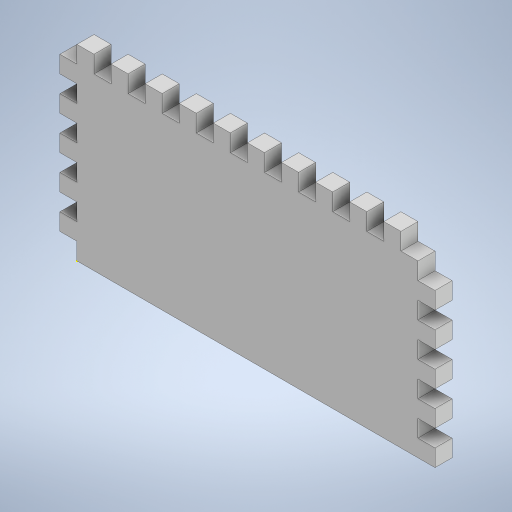
# Autodesk Inventor part: frontbackside
Saved by Autodesk Inventor 2024 (Build 280153000, 153)
## iProperties
Created: 2024-04-15
Part Number: frontbackside
Material: Generic
Document SubType Name: Modeling
Designer: srika
Density: 1 g/cm^3
Appearance: Default
Author: srika
Autodesk Inventor part; units mm, degrees
ref_plane "YZ Plane" through (0, 0, 0) normal (1, 0, 0) x (0, 1, 0)
ref_plane "XZ Plane" through (0, 0, 0) normal (0, 1, 0) x (-1, 0, 0)
ref_plane "XY Plane" through (0, 0, 0) normal (0, 0, 1) x (1, 0, 0)
sketch "Sketch1" plane through (0, 0, 0) normal (0, 0, 1) x (1, 0, 0)
  point P0 (0, 0)
sketch "Sketch2" plane through (0, 0, 0) normal (0, 0, 1) x (1, 0, 0)
  line L0 (0, 0) -> (5, 0)
  line L1 (5, 0) -> (5, 5)
  line L2 (5, 5) -> (0, 5)
  line L3 (0, 5) -> (0, 0)
  line L4 (5, 5) -> (105, 5)
  line L5 (105, 5) -> (105, 55)
  line L6 (105, 55) -> (5, 55)
  line L7 (5, 55) -> (5, 5)
  line L8 (105, 55) -> (110, 55)
  line L9 (110, 55) -> (110, 60)
  line L10 (110, 60) -> (105, 60)
  line L11 (105, 60) -> (105, 55)
  line L12 (100, 60) -> (95, 60)
  line L13 (100, 55) -> (100, 60)
  line L14 (95, 60) -> (95, 55)
  line L15 (90, 60) -> (85, 60)
  line L16 (90, 55) -> (90, 60)
  line L17 (85, 60) -> (85, 55)
  line L18 (80, 60) -> (75, 60)
  line L19 (80, 55) -> (80, 60)
  line L20 (75, 60) -> (75, 55)
  line L21 (70, 60) -> (65, 60)
  line L22 (70, 55) -> (70, 60)
  line L23 (65, 60) -> (65, 55)
  line L24 (60, 60) -> (55, 60)
  line L25 (60, 55) -> (60, 60)
  line L26 (55, 60) -> (55, 55)
  line L27 (50, 60) -> (45, 60)
  line L28 (50, 55) -> (50, 60)
  line L29 (45, 60) -> (45, 55)
  line L30 (40, 60) -> (35, 60)
  line L31 (40, 55) -> (40, 60)
  line L32 (35, 60) -> (35, 55)
  line L33 (30, 60) -> (25, 60)
  line L34 (30, 55) -> (30, 60)
  line L35 (25, 60) -> (25, 55)
  line L36 (20, 60) -> (15, 60)
  line L37 (20, 55) -> (20, 60)
  line L38 (15, 60) -> (15, 55)
  line L39 (10, 60) -> (5, 60)
  line L40 (10, 55) -> (10, 60)
  line L41 (5, 60) -> (5, 55)
  line L42 (105, 50) -> (105, 45)
  line L43 (110, 45) -> (110, 50)
  line L44 (110, 50) -> (105, 50)
  line L45 (105, 45) -> (110, 45)
  line L46 (105, 40) -> (105, 35)
  line L47 (110, 35) -> (110, 40)
  line L48 (110, 40) -> (105, 40)
  line L49 (105, 35) -> (110, 35)
  line L50 (105, 30) -> (105, 25)
  line L51 (110, 25) -> (110, 30)
  line L52 (110, 30) -> (105, 30)
  line L53 (105, 25) -> (110, 25)
  line L54 (105, 20) -> (105, 15)
  line L55 (110, 15) -> (110, 20)
  line L56 (110, 20) -> (105, 20)
  line L57 (105, 15) -> (110, 15)
  line L58 (105, 10) -> (105, 5)
  line L59 (110, 5) -> (110, 10)
  line L60 (110, 10) -> (105, 10)
  line L61 (105, 5) -> (110, 5)
  line L62 (0, 10) -> (5, 10)
  line L63 (5, 10) -> (5, 15)
  line L64 (5, 15) -> (0, 15)
  line L65 (0, 15) -> (0, 10)
  line L66 (0, 20) -> (5, 20)
  line L67 (5, 20) -> (5, 25)
  line L68 (5, 25) -> (0, 25)
  line L69 (0, 25) -> (0, 20)
  line L70 (0, 30) -> (5, 30)
  line L71 (5, 30) -> (5, 35)
  line L72 (5, 35) -> (0, 35)
  line L73 (0, 35) -> (0, 30)
  line L74 (0, 40) -> (5, 40)
  line L75 (5, 40) -> (5, 45)
  line L76 (5, 45) -> (0, 45)
  line L77 (0, 45) -> (0, 40)
  line L78 (0, 50) -> (5, 50)
  line L79 (5, 50) -> (5, 55)
  line L80 (5, 55) -> (0, 55)
  line L81 (0, 55) -> (0, 50)
  line L82 (15, 5) -> (10, 5)
  line L83 (10, 0) -> (15, 0)
  line L84 (15, 0) -> (15, 5)
  line L85 (10, 5) -> (10, 0)
  line L86 (25, 5) -> (20, 5)
  line L87 (20, 0) -> (25, 0)
  line L88 (25, 0) -> (25, 5)
  line L89 (20, 5) -> (20, 0)
  line L90 (35, 5) -> (30, 5)
  line L91 (30, 0) -> (35, 0)
  line L92 (35, 0) -> (35, 5)
  line L93 (30, 5) -> (30, 0)
  line L94 (45, 5) -> (40, 5)
  line L95 (40, 0) -> (45, 0)
  line L96 (45, 0) -> (45, 5)
  line L97 (40, 5) -> (40, 0)
  line L98 (55, 5) -> (50, 5)
  line L99 (50, 0) -> (55, 0)
  line L100 (55, 0) -> (55, 5)
  line L101 (50, 5) -> (50, 0)
  line L102 (65, 5) -> (60, 5)
  line L103 (60, 0) -> (65, 0)
  line L104 (65, 0) -> (65, 5)
  line L105 (60, 5) -> (60, 0)
  line L106 (75, 5) -> (70, 5)
  line L107 (70, 0) -> (75, 0)
  line L108 (75, 0) -> (75, 5)
  line L109 (70, 5) -> (70, 0)
  line L110 (85, 5) -> (80, 5)
  line L111 (80, 0) -> (85, 0)
  line L112 (85, 0) -> (85, 5)
  line L113 (80, 5) -> (80, 0)
  line L114 (95, 5) -> (90, 5)
  line L115 (90, 0) -> (95, 0)
  line L116 (95, 0) -> (95, 5)
  line L117 (90, 5) -> (90, 0)
  line L118 (105, 5) -> (100, 5)
  line L119 (100, 0) -> (105, 0)
  line L120 (105, 0) -> (105, 5)
  line L121 (100, 5) -> (100, 0)
  dimension "d0" = 5
  dimension "d1" = 5
  dimension "d4" = 5
  dimension "d5" = 5
  dimension "d8" = 10
  dimension "d15" = 10
  dimension "d22" = 10
  dimension "d29" = 10
  constraints: 242 end point, 40 horizontal alignment, 25 parallel, 10 collinear, 5 horizontal, 3 perpendicular, 2 vertical, 163 other
  measures "d0" distance of L2.end L1.end
  measures "d1" distance of L1.end L0.end
  measures "d4" distance of L10.end L9.end
  measures "d5" distance of L9.end L8.end
  measures "d8" distance of L9.end L12.start
  measures "d15" distance of L5.end L42.end
  measures "d22" distance of L1.end L63.end
  measures "d29" distance of L2.end L82.end
sketch "Sketch3" plane through (0, 0, 0) normal (0, 0, 1) x (1, 0, 0)
  point P0 (0, 0)
extrude "Extrusion1" add sketch "Sketch2" along normal blind 5 contours L7 L6 L5 L4 | L62 L65 L64 L7 | L66 L69 L68 L7 | L70 L73 L72 L7 | L74 L77 L76 L7 | L78 L81 L80 L7 | L41 L39 L40 L6 | L38 L36 L37 L6 | L35 L33 L34 L6 | L32 L30 L31 L6 | L29 L27 L28 L6 | L5 L60 L59 L61 | L26 L24 L25 L6 | L5 L56 L55 L57 | L23 L21 L22 L6 | L5 L52 L51 L53 | L20 L18 L19 L6 | L5 L48 L47 L49 | L17 L15 L16 L6 | L5 L44 L43 L45 | L14 L12 L13 L6
body "Solid1"
